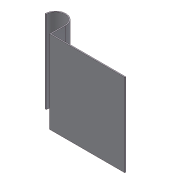
# Autodesk Inventor part: SpaceQuest_interconnect_2
Saved by Autodesk Inventor 2014 SP1 (Build 180222100, 222)
## iProperties
Created: 2013-06-08
Part Number: SpaceQuest_interconnect_2
Material: Stainless Steel
Document SubType Name: Modeling
Designer: Robert Davis
Mass: 0.0072023 g
Surface Area: 0.365006 cm^2
Volume: 0.000891374 cm^3
Density: 8.08 g/cm^3
Appearance: Steel
Author: Robert Davis
Autodesk Inventor part; units mm, degrees
ref_plane "YZ Plane" through (0, 0, 0) normal (1, 0, 0) x (0, 1, 0)
ref_plane "XZ Plane" through (0, 0, 0) normal (0, 1, 0) x (-1, 0, 0)
ref_plane "XY Plane" through (0, 0, 0) normal (0, 0, 1) x (1, 0, 0)
sketch "Sketch1" plane through (0, 0, 0) normal (0, 0, 1) x (1, 0, 0)
  line L0 (0, 0) -> (-3.6, 0)
  line L1 (-3.6, 0) -> (-3.6, 0.7)
  arc A0 (-3.6, 0.7) -> (-4.6, 0.7) centre (-4.1, 0.7) ccw
  arc A1 (-3.65, 0.7) -> (-4.55, 0.7) centre (-4.1, 0.7) ccw
  line L2 (-3.65, 0.7) -> (-3.65, -0.05)
  line L3 (-3.65, -0.05) -> (0, -0.05)
  line L4 (-4.55, 0.7) -> (-4.6, 0.7)
  line L5 (0, -0.05) -> (0, 0)
  dimension "d1" = 0.5
  dimension "d2" = 0.7
  dimension "d3" = 4.6
  dimension "d4" = 0.05
  constraints: 12 end point, 4 point on circle, 2 centre point, 2 horizontal, 2 vertical, 1 coincident, 1 point on line, 1 tangent, 2 other
  measures "d1" radius of A0
  measures "d2" distance of L0.end L1.end
  measures "d3" horizontal distance of L4.end point (0, 0)
  measures "d4" distance between parallel lines of L3 L0
extrude "Extrusion1" add sketch "Sketch1" along normal mid plane 4
equation "\"BendRadius\" = Thickness"
equation "\"BendReliefWidth\" = Thickness"
equation "\"BendReliefDepth\" = 0.5 * Thickness"
equation "\"CornerReliefSize\" = 4 * Thickness"
equation "\"MinimumRemnant\" = 2 * Thickness"
equation "\"TransitionRadius\" = BendRadius"
equation "\"JacobiRadiusSize\" = Thickness"
equation "\"GapSize\" = Thickness"
equation "\"Thickness\" = 0.5"
body "Solid1"
